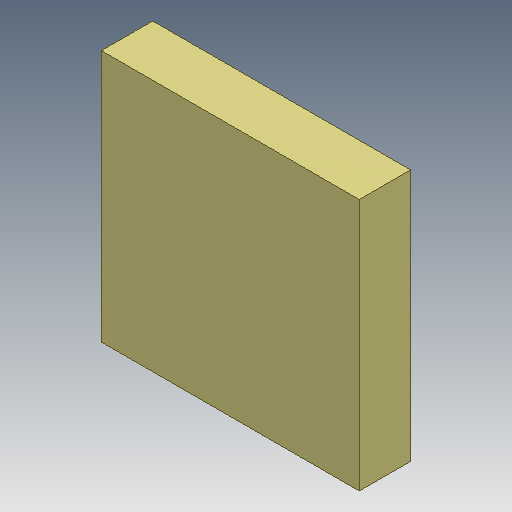
# Autodesk Inventor part: GREEN
Saved by Autodesk Inventor 2017 (Build 210142000, 142)
## iProperties
Part Number: GREEN
Material: Generisch
Document SubType Name: Modeling
Designer: Werkstatt
Density: 1 g/cm^3
Appearance: LED-0603, GREEN
Author: Werkstatt
Autodesk Inventor part; units mm, degrees
ref_plane "YZ Plane" through (0, 0, 0) normal (1, 0, 0) x (0, 1, 0)
ref_plane "XZ Plane" through (0, 0, 0) normal (0, 1, 0) x (-1, 0, 0)
ref_plane "XY Plane" through (0, 0, 0) normal (0, 0, 1) x (1, 0, 0)
sketch "LED-0603, GREEN_11" plane through (0, 0, 0) normal (0, 0, 1) x (1, 0, 0)
  line L0 (-0.46, 0.2716) -> (0.5616, 0.2716)
  line L1 (0.5616, 0.2716) -> (0.5616, 0.0684)
  line L2 (0.5616, 0.0684) -> (-0.46, 0.0684)
  line L3 (-0.46, 0.0684) -> (-0.46, 0.2716)
  constraints: 8 end point
extrude "Extrusion1" add sketch "LED-0603, GREEN_11" along normal blind 1
